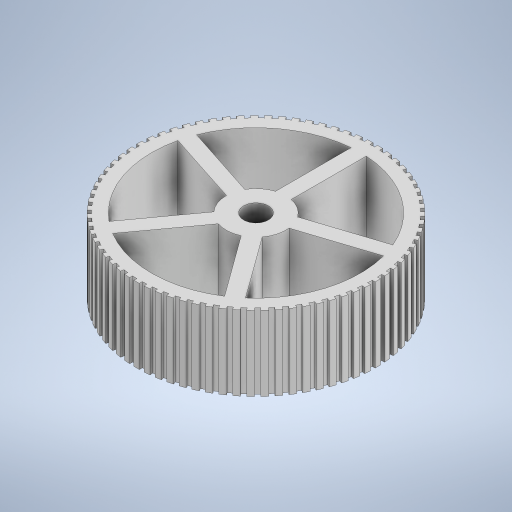
# Autodesk Inventor part: wheel
Saved by Autodesk Inventor 2023 (Build 270158000, 158)
## iProperties
Created: 2022-10-31
Part Number: wheel
Material: Generic
Document SubType Name: Modeling
Designer: neera
Density: 1 g/cm^3
Appearance: Default
Author: neera
Autodesk Inventor part; units mm, degrees
ref_plane "YZ Plane" through (0, 0, 0) normal (1, 0, 0) x (0, 1, 0)
ref_plane "XZ Plane" through (0, 0, 0) normal (0, 1, 0) x (-1, 0, 0)
ref_plane "XY Plane" through (0, 0, 0) normal (0, 0, 1) x (1, 0, 0)
sketch "Sketch1" plane through (0, 0, 0) normal (0, 1, 0) x (-1, 0, 0)
  circle A0 centre (0, 0) radius 40
  dimension "d0" = 80
  constraints: 1 centre point, 1 coincident
  measures "d0" diameter of A0
extrude "Extrusion1" add sketch "Sketch1" along normal blind 25
sketch "Sketch3" plane through (0, 25, 0) normal (0, 1, 0) x (1, 0, 0)
  circle A0 centre (0, 0) radius 35
  line L0 (0, 0) -> (57.5, 0) construction
  circle A1 centre (0, 0) radius 10
  line L1 (2, 9.798) -> (2, 34.9428)
  line L2 (-3, 9.5394) -> (-3, 34.8712)
  line L3 (-8.7004, 4.9298) -> (-32.6146, 12.7)
  line L4 (-9.9996, 0.0947) -> (-34.0915, 7.9226)
  line L5 (-7.3771, -6.7511) -> (-22.1569, -27.0938)
  line L6 (-3.1801, -9.4809) -> (-18.0697, -29.9747)
  line L7 (4.1411, -9.1023) -> (18.9208, -29.4449)
  line L8 (8.0342, -5.9542) -> (22.9238, -26.448)
  line L9 (9.9364, 1.1256) -> (33.8506, 8.8958)
  line L10 (8.1454, 5.801) -> (32.2374, 13.629)
  point P0 (33.8506, 8.8958)
  point P1 (9.9364, 1.1256)
  point P2 (8.0342, -5.9542)
  point P3 (22.9238, -26.448)
  point P4 (4.1411, -9.1023)
  point P5 (-3.1801, -9.4809)
  point P6 (-7.3771, -6.7511)
  point P7 (-9.9996, 0.0947)
  point P8 (-34.0915, 7.9226)
  point P9 (-32.6146, 12.7)
  point P10 (-8.7004, 4.9298)
  point P11 (8.1454, 5.801)
  dimension "d6" = 70
  dimension "d8" = 20
  dimension "d9" = 2
  dimension "d10" = 3
  dimension "d13" = 360
  constraints: 22 end point, 4 point on circle, 2 centre point, 2 coincident, 2 vertical, 1 horizontal, 31 other
  measures "d6" diameter of A0
  measures "d8" diameter of A1
  measures "d9" horizontal distance of point (0, 0) L1.start
  measures "d10" horizontal distance of point (0, 0) L2.start
extrude "Extrusion3" cut sketch "Sketch3" against normal blind 40 contours A0 L8 A1 L9 | L10 A1 L1 A0 | A0 L6 A1 L7 | L2 A1 L3 A0 | A0 L4 A1 L5
sketch "Sketch9" plane through (0, 0, 0) normal (0, -1, 0) x (1, 0, 0)
  line L0 (0.75, -41) -> (-0.75, -41)
  line L1 (-0.75, -41) -> (-0.75, -39)
  line L2 (-0.75, -39) -> (0.75, -39)
  line L3 (0.75, -39) -> (0.75, -41)
  circle A0 centre (0, 0) radius 40 projected
  line L4 (0.75, -41) -> (-0.75, -39) construction
  line L5 (-0.75, -41) -> (0.75, -39) construction
  line L6 (2.5161, -38.926) -> (4.0108, -38.8005)
  line L7 (4.0108, -38.8005) -> (4.1782, -40.7934)
  line L8 (2.6834, -40.919) -> (2.5161, -38.926)
  line L9 (4.1782, -40.7934) -> (2.6834, -40.919)
  line L10 (5.7645, -38.5789) -> (7.2435, -38.3288)
  line L11 (7.2435, -38.3288) -> (7.577, -40.3008)
  line L12 (6.098, -40.5509) -> (5.7645, -38.5789)
  line L13 (7.577, -40.3008) -> (6.098, -40.5509)
  line L14 (8.9725, -37.9613) -> (10.4253, -37.5882)
  line L15 (10.4253, -37.5882) -> (10.9227, -39.5254)
  line L16 (9.4698, -39.8984) -> (8.9725, -37.9613)
  line L17 (10.9227, -39.5254) -> (9.4698, -39.8984)
  line L18 (12.1175, -37.0773) -> (13.5341, -36.584)
  line L19 (13.5341, -36.584) -> (14.1918, -38.4728)
  line L20 (12.7753, -38.9661) -> (12.1175, -37.0773)
  line L21 (14.1918, -38.4728) -> (12.7753, -38.9661)
  line L22 (15.1776, -35.9333) -> (16.5479, -35.3232)
  line L23 (16.5479, -35.3232) -> (17.3614, -37.1503)
  line L24 (15.991, -37.7604) -> (15.1776, -35.9333)
  line L25 (17.3614, -37.1503) -> (15.991, -37.7604)
  line L26 (18.1312, -34.5373) -> (19.4456, -33.8146)
  line L27 (19.4456, -33.8146) -> (20.4091, -35.5673)
  line L28 (19.0947, -36.2899) -> (18.1312, -34.5373)
  line L29 (20.4091, -35.5673) -> (19.0947, -36.2899)
  line L30 (20.9576, -32.899) -> (22.207, -32.0689)
  line L31 (22.207, -32.0689) -> (23.3137, -33.7347)
  line L32 (22.0644, -34.5648) -> (20.9576, -32.899)
  line L33 (23.3137, -33.7347) -> (22.0644, -34.5648)
  line L34 (23.637, -31.0299) -> (24.8125, -30.0982)
  line L35 (24.8125, -30.0982) -> (26.0548, -31.6656)
  line L36 (24.8793, -32.5973) -> (23.637, -31.0299)
  line L37 (26.0548, -31.6656) -> (24.8793, -32.5973)
  line L38 (26.1506, -28.9432) -> (27.2441, -27.9164)
  line L39 (27.2441, -27.9164) -> (28.6132, -29.3743)
  line L40 (27.5197, -30.4011) -> (26.1506, -28.9432)
  line L41 (28.6132, -29.3743) -> (27.5197, -30.4011)
  line L42 (28.4808, -26.6535) -> (29.4845, -25.5387)
  line L43 (29.4845, -25.5387) -> (30.9708, -26.877)
  line L44 (29.9671, -27.9917) -> (28.4808, -26.6535)
  line L45 (30.9708, -26.877) -> (29.9671, -27.9917)
  line L46 (30.6112, -24.1768) -> (31.5181, -22.982)
  line L47 (31.5181, -22.982) -> (33.1112, -24.1912)
  line L48 (32.2043, -25.386) -> (30.6112, -24.1768)
  line L49 (33.1112, -24.1912) -> (32.2043, -25.386)
  line L50 (32.5269, -21.5305) -> (33.3307, -20.264)
  line L51 (33.3307, -20.264) -> (35.0193, -21.3357)
  line L52 (34.2156, -22.6021) -> (32.5269, -21.5305)
  line L53 (35.0193, -21.3357) -> (34.2156, -22.6021)
  line L54 (34.2145, -18.7332) -> (34.9094, -17.4039)
  line L55 (34.9094, -17.4039) -> (36.6818, -18.3305)
  line L56 (35.9869, -19.6598) -> (34.2145, -18.7332)
  line L57 (36.6818, -18.3305) -> (35.9869, -19.6598)
  line L58 (35.662, -15.8045) -> (36.2433, -14.4217)
  line L59 (36.2433, -14.4217) -> (38.087, -15.1967)
  line L60 (37.5058, -16.5795) -> (35.662, -15.8045)
  line L61 (38.087, -15.1967) -> (37.5058, -16.5795)
  line L62 (36.8594, -12.765) -> (37.323, -11.3384)
  line L63 (37.323, -11.3384) -> (39.2251, -11.9564)
  line L64 (38.7616, -13.383) -> (36.8594, -12.765)
  line L65 (39.2251, -11.9564) -> (38.7616, -13.383)
  line L66 (37.7983, -9.6359) -> (38.1408, -8.1755)
  line L67 (38.1408, -8.1755) -> (40.088, -8.6322)
  line L68 (39.7455, -10.0926) -> (37.7983, -9.6359)
  line L69 (40.088, -8.6322) -> (39.7455, -10.0926)
  line L70 (38.4721, -6.4392) -> (38.6912, -4.9553)
  line L71 (38.6912, -4.9553) -> (40.6697, -5.2474)
  line L72 (40.4506, -6.7314) -> (38.4721, -6.4392)
  line L73 (40.6697, -5.2474) -> (40.4506, -6.7314)
  line L74 (38.8759, -3.1974) -> (38.9701, -1.7003)
  line L75 (38.9701, -1.7003) -> (40.9662, -1.8259)
  line L76 (40.872, -3.3229) -> (38.8759, -3.1974)
  line L77 (40.9662, -1.8259) -> (40.872, -3.3229)
  line L78 (39.0072, 0.0669) -> (38.9757, 1.5666)
  line L79 (38.9757, 1.5666) -> (40.9753, 1.6085)
  line L80 (41.0067, 0.1088) -> (39.0072, 0.0669)
  line L81 (40.9753, 1.6085) -> (41.0067, 0.1088)
  line L82 (38.8648, 3.3307) -> (38.708, 4.8225)
  line L83 (38.708, 4.8225) -> (40.697, 5.0316)
  line L84 (40.8538, 3.5398) -> (38.8648, 3.3307)
  line L85 (40.697, 5.0316) -> (40.8538, 3.5398)
  line L86 (38.4497, 6.5712) -> (38.1687, 8.0446)
  line L87 (38.1687, 8.0446) -> (40.1332, 8.4193)
  line L88 (40.4143, 6.9459) -> (38.4497, 6.5712)
  line L89 (40.1332, 8.4193) -> (40.4143, 6.9459)
  line L90 (37.765, 9.7655) -> (37.3617, 11.2102)
  line L91 (37.3617, 11.2102) -> (39.288, 11.7481)
  line L92 (39.6914, 10.3033) -> (37.765, 9.7655)
  line L93 (39.288, 11.7481) -> (39.6914, 10.3033)
  line L94 (36.8154, 12.8913) -> (36.2926, 14.2973)
  line L95 (36.2926, 14.2973) -> (38.1671, 14.9944)
  line L96 (38.69, 13.5885) -> (36.8154, 12.8913)
  line L97 (38.1671, 14.9944) -> (38.69, 13.5885)
  line L98 (35.6076, 15.9268) -> (34.9689, 17.284)
  line L99 (34.9689, 17.284) -> (36.7786, 18.1356)
  line L100 (37.4172, 16.7783) -> (35.6076, 15.9268)
  line L101 (36.7786, 18.1356) -> (37.4172, 16.7783)
  line L102 (34.15, 18.8505) -> (33.4, 20.1495)
  line L103 (33.4, 20.1495) -> (35.132, 21.1495)
  line L104 (35.882, 19.8505) -> (34.15, 18.8505)
  line L105 (35.132, 21.1495) -> (35.882, 19.8505)
  line L106 (32.4529, 21.642) -> (31.5968, 22.8737)
  line L107 (31.5968, 22.8737) -> (33.2391, 24.0151)
  line L108 (34.0952, 22.7834) -> (32.4529, 21.642)
  line L109 (33.2391, 24.0151) -> (34.0952, 22.7834)
  line L110 (30.5281, 24.2817) -> (29.5719, 25.4374)
  line L111 (29.5719, 25.4374) -> (31.113, 26.7123)
  line L112 (32.0691, 25.5565) -> (30.5281, 24.2817)
  line L113 (31.113, 26.7123) -> (32.0691, 25.5565)
  line L114 (28.3892, 26.751) -> (27.3397, 27.8227)
  line L115 (27.3397, 27.8227) -> (28.7686, 29.2221)
  line L116 (29.8181, 28.1503) -> (28.3892, 26.751)
  line L117 (28.7686, 29.2221) -> (29.8181, 28.1503)
  line L118 (26.0511, 29.0327) -> (24.9157, 30.0129)
  line L119 (24.9157, 30.0129) -> (26.2225, 31.5269)
  line L120 (27.358, 30.5467) -> (26.0511, 29.0327)
  line L121 (26.2225, 31.5269) -> (27.358, 30.5467)
  line L122 (23.5304, 31.1108) -> (22.3169, 31.9925)
  line L123 (22.3169, 31.9925) -> (23.4924, 33.6105)
  line L124 (24.706, 32.7289) -> (23.5304, 31.1108)
  line L125 (23.4924, 33.6105) -> (24.706, 32.7289)
  line L126 (20.8446, 32.9707) -> (19.5615, 33.7477)
  line L127 (19.5615, 33.7477) -> (20.5976, 35.4585)
  line L128 (21.8806, 34.6814) -> (20.8446, 32.9707)
  line L129 (20.5976, 35.4585) -> (21.8806, 34.6814)
  line L130 (18.0126, 34.5993) -> (16.669, 35.2662)
  line L131 (16.669, 35.2662) -> (17.5583, 37.0577)
  line L132 (18.9018, 36.3907) -> (18.0126, 34.5993)
  line L133 (17.5583, 37.0577) -> (18.9018, 36.3907)
  line L134 (15.0542, 35.9852) -> (13.6595, 36.5374)
  line L135 (13.6595, 36.5374) -> (14.3958, 38.3969)
  line L136 (15.7904, 37.8447) -> (15.0542, 35.9852)
  line L137 (14.3958, 38.3969) -> (15.7904, 37.8447)
  line L138 (11.9902, 37.1187) -> (10.5543, 37.5522)
  line L139 (10.5543, 37.5522) -> (11.1323, 39.4669)
  line L140 (12.5683, 39.0333) -> (11.9902, 37.1187)
  line L141 (11.1323, 39.4669) -> (12.5683, 39.0333)
  line L142 (8.8422, 37.9918) -> (7.3749, 38.3037)
  line L143 (7.3749, 38.3037) -> (7.7908, 40.26)
  line L144 (9.258, 39.9481) -> (8.8422, 37.9918)
  line L145 (7.7908, 40.26) -> (9.258, 39.9481)
  line L146 (5.6321, 38.5985) -> (4.1439, 38.7865)
  line L147 (4.1439, 38.7865) -> (4.3946, 40.7707)
  line L148 (5.8827, 40.5827) -> (5.6321, 38.5985)
  line L149 (4.3946, 40.7707) -> (5.8827, 40.5827)
  line L150 (2.3825, 38.9344) -> (0.8838, 38.9972)
  line L151 (0.8838, 38.9972) -> (0.9676, 40.9954)
  line L152 (2.4662, 40.9326) -> (2.3825, 38.9344)
  line L153 (0.9676, 40.9954) -> (2.4662, 40.9326)
  line L154 (-0.8838, 38.9972) -> (-2.3825, 38.9344)
  line L155 (-2.3825, 38.9344) -> (-2.4662, 40.9326)
  line L156 (-0.9676, 40.9954) -> (-0.8838, 38.9972)
  line L157 (-2.4662, 40.9326) -> (-0.9676, 40.9954)
  line L158 (-4.1439, 38.7865) -> (-5.6321, 38.5985)
  line L159 (-5.6321, 38.5985) -> (-5.8827, 40.5827)
  line L160 (-4.3946, 40.7707) -> (-4.1439, 38.7865)
  line L161 (-5.8827, 40.5827) -> (-4.3946, 40.7707)
  line L162 (-7.3749, 38.3037) -> (-8.8422, 37.9918)
  line L163 (-8.8422, 37.9918) -> (-9.258, 39.9481)
  line L164 (-7.7908, 40.26) -> (-7.3749, 38.3037)
  line L165 (-9.258, 39.9481) -> (-7.7908, 40.26)
  line L166 (-10.5543, 37.5522) -> (-11.9902, 37.1187)
  line L167 (-11.9902, 37.1187) -> (-12.5683, 39.0333)
  line L168 (-11.1323, 39.4669) -> (-10.5543, 37.5522)
  line L169 (-12.5683, 39.0333) -> (-11.1323, 39.4669)
  line L170 (-13.6595, 36.5374) -> (-15.0542, 35.9852)
  line L171 (-15.0542, 35.9852) -> (-15.7904, 37.8447)
  line L172 (-14.3958, 38.3969) -> (-13.6595, 36.5374)
  line L173 (-15.7904, 37.8447) -> (-14.3958, 38.3969)
  line L174 (-16.669, 35.2662) -> (-18.0126, 34.5993)
  line L175 (-18.0126, 34.5993) -> (-18.9018, 36.3907)
  line L176 (-17.5583, 37.0577) -> (-16.669, 35.2662)
  line L177 (-18.9018, 36.3907) -> (-17.5583, 37.0577)
  line L178 (-19.5615, 33.7477) -> (-20.8446, 32.9707)
  line L179 (-20.8446, 32.9707) -> (-21.8806, 34.6814)
  line L180 (-20.5976, 35.4585) -> (-19.5615, 33.7477)
  line L181 (-21.8806, 34.6814) -> (-20.5976, 35.4585)
  line L182 (-22.3169, 31.9925) -> (-23.5304, 31.1108)
  line L183 (-23.5304, 31.1108) -> (-24.706, 32.7289)
  line L184 (-23.4924, 33.6105) -> (-22.3169, 31.9925)
  line L185 (-24.706, 32.7289) -> (-23.4924, 33.6105)
  line L186 (-24.9157, 30.0129) -> (-26.0511, 29.0327)
  line L187 (-26.0511, 29.0327) -> (-27.358, 30.5467)
  line L188 (-26.2225, 31.5269) -> (-24.9157, 30.0129)
  line L189 (-27.358, 30.5467) -> (-26.2225, 31.5269)
  line L190 (-27.3397, 27.8227) -> (-28.3892, 26.751)
  line L191 (-28.3892, 26.751) -> (-29.8181, 28.1503)
  line L192 (-28.7686, 29.2221) -> (-27.3397, 27.8227)
  line L193 (-29.8181, 28.1503) -> (-28.7686, 29.2221)
  line L194 (-29.5719, 25.4374) -> (-30.5281, 24.2817)
  line L195 (-30.5281, 24.2817) -> (-32.0691, 25.5565)
  line L196 (-31.113, 26.7123) -> (-29.5719, 25.4374)
  line L197 (-32.0691, 25.5565) -> (-31.113, 26.7123)
  line L198 (-31.5968, 22.8737) -> (-32.4529, 21.642)
  line L199 (-32.4529, 21.642) -> (-34.0952, 22.7834)
  line L200 (-33.2391, 24.0151) -> (-31.5968, 22.8737)
  line L201 (-34.0952, 22.7834) -> (-33.2391, 24.0151)
  line L202 (-33.4, 20.1495) -> (-34.15, 18.8505)
  line L203 (-34.15, 18.8505) -> (-35.882, 19.8505)
  line L204 (-35.132, 21.1495) -> (-33.4, 20.1495)
  line L205 (-35.882, 19.8505) -> (-35.132, 21.1495)
  line L206 (-34.9689, 17.284) -> (-35.6076, 15.9268)
  line L207 (-35.6076, 15.9268) -> (-37.4172, 16.7783)
  line L208 (-36.7786, 18.1356) -> (-34.9689, 17.284)
  line L209 (-37.4172, 16.7783) -> (-36.7786, 18.1356)
  line L210 (-36.2926, 14.2973) -> (-36.8154, 12.8913)
  line L211 (-36.8154, 12.8913) -> (-38.69, 13.5885)
  line L212 (-38.1671, 14.9944) -> (-36.2926, 14.2973)
  line L213 (-38.69, 13.5885) -> (-38.1671, 14.9944)
  line L214 (-37.3617, 11.2102) -> (-37.765, 9.7655)
  line L215 (-37.765, 9.7655) -> (-39.6914, 10.3033)
  line L216 (-39.288, 11.7481) -> (-37.3617, 11.2102)
  line L217 (-39.6914, 10.3033) -> (-39.288, 11.7481)
  line L218 (-38.1687, 8.0446) -> (-38.4497, 6.5712)
  line L219 (-38.4497, 6.5712) -> (-40.4143, 6.9459)
  line L220 (-40.1332, 8.4193) -> (-38.1687, 8.0446)
  line L221 (-40.4143, 6.9459) -> (-40.1332, 8.4193)
  line L222 (-38.708, 4.8225) -> (-38.8648, 3.3307)
  line L223 (-38.8648, 3.3307) -> (-40.8538, 3.5398)
  line L224 (-40.697, 5.0316) -> (-38.708, 4.8225)
  line L225 (-40.8538, 3.5398) -> (-40.697, 5.0316)
  line L226 (-38.9757, 1.5666) -> (-39.0072, 0.0669)
  line L227 (-39.0072, 0.0669) -> (-41.0067, 0.1088)
  line L228 (-40.9753, 1.6085) -> (-38.9757, 1.5666)
  line L229 (-41.0067, 0.1088) -> (-40.9753, 1.6085)
  line L230 (-38.9701, -1.7003) -> (-38.8759, -3.1974)
  line L231 (-38.8759, -3.1974) -> (-40.872, -3.3229)
  line L232 (-40.9662, -1.8259) -> (-38.9701, -1.7003)
  line L233 (-40.872, -3.3229) -> (-40.9662, -1.8259)
  line L234 (-38.6912, -4.9553) -> (-38.4721, -6.4392)
  line L235 (-38.4721, -6.4392) -> (-40.4506, -6.7314)
  line L236 (-40.6697, -5.2474) -> (-38.6912, -4.9553)
  line L237 (-40.4506, -6.7314) -> (-40.6697, -5.2474)
  line L238 (-38.1408, -8.1755) -> (-37.7983, -9.6359)
  line L239 (-37.7983, -9.6359) -> (-39.7455, -10.0926)
  line L240 (-40.088, -8.6322) -> (-38.1408, -8.1755)
  line L241 (-39.7455, -10.0926) -> (-40.088, -8.6322)
  line L242 (-37.323, -11.3384) -> (-36.8594, -12.765)
  line L243 (-36.8594, -12.765) -> (-38.7616, -13.383)
  line L244 (-39.2251, -11.9564) -> (-37.323, -11.3384)
  line L245 (-38.7616, -13.383) -> (-39.2251, -11.9564)
  line L246 (-36.2433, -14.4217) -> (-35.662, -15.8045)
  line L247 (-35.662, -15.8045) -> (-37.5058, -16.5795)
  line L248 (-38.087, -15.1967) -> (-36.2433, -14.4217)
  line L249 (-37.5058, -16.5795) -> (-38.087, -15.1967)
  line L250 (-34.9094, -17.4039) -> (-34.2145, -18.7332)
  line L251 (-34.2145, -18.7332) -> (-35.9869, -19.6598)
  line L252 (-36.6818, -18.3305) -> (-34.9094, -17.4039)
  line L253 (-35.9869, -19.6598) -> (-36.6818, -18.3305)
  line L254 (-33.3307, -20.264) -> (-32.5269, -21.5305)
  line L255 (-32.5269, -21.5305) -> (-34.2156, -22.6021)
  line L256 (-35.0193, -21.3357) -> (-33.3307, -20.264)
  line L257 (-34.2156, -22.6021) -> (-35.0193, -21.3357)
  line L258 (-31.5181, -22.982) -> (-30.6112, -24.1768)
  line L259 (-30.6112, -24.1768) -> (-32.2043, -25.386)
  line L260 (-33.1112, -24.1912) -> (-31.5181, -22.982)
  line L261 (-32.2043, -25.386) -> (-33.1112, -24.1912)
  line L262 (-29.4845, -25.5387) -> (-28.4808, -26.6535)
  line L263 (-28.4808, -26.6535) -> (-29.9671, -27.9917)
  line L264 (-30.9708, -26.877) -> (-29.4845, -25.5387)
  line L265 (-29.9671, -27.9917) -> (-30.9708, -26.877)
  line L266 (-27.2441, -27.9164) -> (-26.1506, -28.9432)
  line L267 (-26.1506, -28.9432) -> (-27.5197, -30.4011)
  line L268 (-28.6132, -29.3743) -> (-27.2441, -27.9164)
  line L269 (-27.5197, -30.4011) -> (-28.6132, -29.3743)
  line L270 (-24.8125, -30.0982) -> (-23.637, -31.0299)
  line L271 (-23.637, -31.0299) -> (-24.8793, -32.5973)
  line L272 (-26.0548, -31.6656) -> (-24.8125, -30.0982)
  line L273 (-24.8793, -32.5973) -> (-26.0548, -31.6656)
  line L274 (-22.207, -32.0689) -> (-20.9576, -32.899)
  line L275 (-20.9576, -32.899) -> (-22.0644, -34.5648)
  line L276 (-23.3137, -33.7347) -> (-22.207, -32.0689)
  line L277 (-22.0644, -34.5648) -> (-23.3137, -33.7347)
  line L278 (-19.4456, -33.8146) -> (-18.1312, -34.5373)
  line L279 (-18.1312, -34.5373) -> (-19.0947, -36.2899)
  line L280 (-20.4091, -35.5673) -> (-19.4456, -33.8146)
  line L281 (-19.0947, -36.2899) -> (-20.4091, -35.5673)
  line L282 (-16.5479, -35.3232) -> (-15.1776, -35.9333)
  line L283 (-15.1776, -35.9333) -> (-15.991, -37.7604)
  line L284 (-17.3614, -37.1503) -> (-16.5479, -35.3232)
  line L285 (-15.991, -37.7604) -> (-17.3614, -37.1503)
  line L286 (-13.5341, -36.584) -> (-12.1175, -37.0773)
  line L287 (-12.1175, -37.0773) -> (-12.7753, -38.9661)
  line L288 (-14.1918, -38.4728) -> (-13.5341, -36.584)
  line L289 (-12.7753, -38.9661) -> (-14.1918, -38.4728)
  line L290 (-10.4253, -37.5882) -> (-8.9725, -37.9613)
  line L291 (-8.9725, -37.9613) -> (-9.4698, -39.8984)
  line L292 (-10.9227, -39.5254) -> (-10.4253, -37.5882)
  line L293 (-9.4698, -39.8984) -> (-10.9227, -39.5254)
  line L294 (-7.2435, -38.3288) -> (-5.7645, -38.5789)
  line L295 (-5.7645, -38.5789) -> (-6.098, -40.5509)
  line L296 (-7.577, -40.3008) -> (-7.2435, -38.3288)
  line L297 (-6.098, -40.5509) -> (-7.577, -40.3008)
  line L298 (-4.0108, -38.8005) -> (-2.5161, -38.926)
  line L299 (-2.5161, -38.926) -> (-2.6834, -40.919)
  line L300 (-4.1782, -40.7934) -> (-4.0108, -38.8005)
  line L301 (-2.6834, -40.919) -> (-4.1782, -40.7934)
  point P0 (0, -40)
  point P1 (-26.7, 29.7844)
  point P2 (-25.5645, 30.7645)
  point P3 (-24.114, 31.9142)
  point P4 (-22.9005, 32.7958)
  point P5 (-21.359, 33.82)
  point P6 (-20.0759, 34.5971)
  point P7 (-12.2772, 38.0693)
  point P8 (-10.8412, 38.5028)
  point P9 (-2.4241, 39.9265)
  point P10 (-0.9254, 39.9893)
  point P11 (0.9254, 39.9893)
  point P12 (2.4241, 39.9265)
  point P13 (4.2684, 39.7716)
  point P14 (5.7565, 39.5836)
  point P15 (7.5814, 39.275)
  point P16 (9.0486, 38.9631)
  point P17 (20.0759, 34.5971)
  point P18 (21.359, 33.82)
  point P19 (25.5645, 30.7645)
  point P20 (26.7, 29.7844)
  dimension "d37" = 1.5
  dimension "d38" = 2
  dimension "d41" = 360
  constraints: 604 end point, 2 midpoint, 2 parallel, 1 horizontal, 1 perpendicular, 603 other
  measures "d37" distance of L1.end L2.end
  measures "d38" distance of L0.end L1.end
extrude "Extrusion9" cut sketch "Sketch9" against normal blind 40 contours L0 L1 A0 L3 | A0 L1 L2 L3 | L8 L6 L7 A0 | A0 L7 L9 L8 | L299 L301 L300 A0 | A0 L300 L298 L299 | L12 L10 L11 A0 | A0 L11 L13 L12 | L295 L297 L296 A0 | A0 L296 L294 L295 | L16 L14 L15 A0 | A0 L15 L17 L16 | L291 L293 L292 A0 | A0 L292 L290 L291 | L20 L18 L19 A0 | A0 L19 L21 L20 | L287 L289 L288 A0 | A0 L288 L286 L287 | L24 L22 L23 A0 | A0 L23 L25 L24 | L283 L285 L284 A0 | A0 L284 L282 L283 | L28 L26 L27 A0 | A0 L27 L29 L28 | L279 L281 L280 A0 | A0 L280 L278 L279 | L32 L30 L31 A0 | A0 L31 L33 L32 | L275 L277 L276 A0 | A0 L276 L274 L275 | L36 L34 L35 A0 | A0 L35 L37 L36 | L271 L273 L272 A0 | A0 L272 L270 L271 | L40 L38 L39 A0 | A0 L39 L41 L40 | L267 L269 L268 A0 | A0 L268 L266 L267 | L44 L42 L43 A0 | A0 L43 L45 L44 | L263 L265 L264 A0 | A0 L264 L262 L263 | L48 L46 L47 A0 | A0 L47 L49 L48 | L259 L261 L260 A0 | A0 L260 L258 L259 | L52 L50 L51 A0 | A0 L51 L53 L52 | L255 L257 L256 A0 | A0 L256 L254 L255 | L56 L54 L55 A0 | A0 L55 L57 L56 | L251 L253 L252 A0 | A0 L252 L250 L251 | L60 L58 L59 A0 | A0 L59 L61 L60 | L247 L249 L248 A0 | A0 L248 L246 L247 | L64 L62 L63 A0 | A0 L63 L65 L64 | L243 L245 L244 A0 | A0 L244 L242 L243 | L68 L66 L67 A0 | A0 L67 L69 L68 | L239 L241 L240 A0 | A0 L240 L238 L239 | L72 L70 L71 A0 | A0 L71 L73 L72 | L235 L237 L236 A0 | A0 L236 L234 L235 | L76 L74 L75 A0 | A0 L75 L77 L76 | L231 L233 L232 A0 | A0 L232 L230 L231 | L227 L229 L228 A0 | A0 L228 L226 L227 | L80 L78 L79 A0 | A0 L79 L81 L80 | L223 L225 L224 A0 | A0 L224 L222 L223 | L84 L82 L83 A0 | A0 L83 L85 L84 | L219 L221 L220 A0 | A0 L220 L218 L219 | L88 L86 L87 A0 | A0 L87 L89 L88 | L215 L217 L216 A0 | A0 L216 L214 L215 | L92 L90 L91 A0 | A0 L91 L93 L92 | L211 L213 L212 A0 | A0 L212 L210 L211 | L96 L94 L95 A0 | A0 L95 L97 L96 | L207 L209 L208 A0 | A0 L208 L206 L207 | L100 L98 L99 A0 | A0 L99 L101 L100 | L203 L205 L204 A0 | A0 L204 L202 L203 | L104 L102 L103 A0 | A0 L103 L105 L104 | L199 L201 L200 A0 | A0 L200 L198 L199 | L108 L106 L107 A0 | A0 L107 L109 L108 | L195 L197 L196 A0 | A0 L196 L194 L195 | L112 L110 L111 A0 | A0 L111 L113 L112 | L191 L193 L192 A0 | A0 L192 L190 L191 | L116 L114 L115 A0 | A0 L115 L117 L116 | L187 L189 L188 A0 | A0 L188 L186 L187 | L120 L118 L119 A0 | A0 L119 L121 L120 | L183 L185 L184 A0 | A0 L184 L182 L183 | L124 L122 L123 A0 | A0 L123 L125 L124 | L179 L181 L180 A0 | A0 L180 L178 L179 | L128 L126 L127 A0 | A0 L127 L129 L128 | L175 L177 L176 A0 | A0 L176 L174 L175 | L132 L130 L131 A0 | A0 L131 L133 L132 | L171 L173 L172 A0 | A0 L172 L170 L171 | L136 L134 L135 A0 | A0 L135 L137 L136 | L167 L169 L168 A0 | A0 L168 L166 L167 | L140 L138 L139 A0 | A0 L139 L141 L140 | L163 L165 L164 A0 | A0 L164 L162 L163 | L144 L142 L143 A0 | A0 L143 L145 L144 | L159 L161 L160 A0 | A0 L160 L158 L159 | L148 L146 L147 A0 | A0 L147 L149 L148 | L155 L157 L156 A0 | A0 L156 L154 L155 | L152 L150 L151 A0 | A0 L151 L153 L152
sketch "Sketch11" plane through (0, 0, 0) normal (0, -1, 0) x (1, 0, 0)
  circle A0 centre (0, 0) radius 4.15
  dimension "d54" = 8.3
  constraints: 1 centre point, 1 coincident
  measures "d54" diameter of A0
extrude "Extrusion11" cut sketch "Sketch11" against normal blind 40
sketch "Sketch16" plane through (0, 0, 0) normal (0, -1, 0) x (1, 0, 0)
  line L0 (4.0992, 7.1) -> (-4.0992, 7.1)
  line L1 (-4.0992, 7.1) -> (-8.1984, 0)
  line L2 (-8.1984, 0) -> (-4.0992, -7.1)
  line L3 (-4.0992, -7.1) -> (4.0992, -7.1)
  line L4 (4.0992, -7.1) -> (8.1984, 0)
  line L5 (8.1984, 0) -> (4.0992, 7.1)
  line L6 (-8.1984, 0) -> (0, 0) construction
  line L7 (0, 0) -> (8.1984, 0) construction
  dimension "d83" = 120
  dimension "d87" = 14.2
  constraints: 16 end point, 10 equal length, 2 horizontal
  measures "d83" angle of L4 L5
  measures "d87" distance between parallel lines of L3 L0
extrude "Extrusion16" cut sketch "Sketch16" against normal blind 2.5
body "Solid1"
